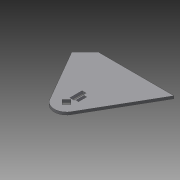
# Autodesk Inventor part: Frame_Lower_Plate_Top
Saved by Autodesk Inventor 2014 (Build 180170000, 170)
## iProperties
Created: 2014-08-25
Part Number: Frame_Lower_Plate_Top
Material: Generic
Document SubType Name: Modeling
Designer: ThatOtherGuy
Density: 1 g/cm^3
Appearance: Default
Author: ThatOtherGuy
Autodesk Inventor part; units mm, degrees
ref_plane "YZ Plane" through (0, 0, 0) normal (1, 0, 0) x (0, 1, 0)
ref_plane "XZ Plane" through (0, 0, 0) normal (0, 1, 0) x (-1, 0, 0)
ref_plane "XY Plane" through (0, 0, 0) normal (0, 0, 1) x (1, 0, 0)
sketch "Sketch1" plane through (0, 0, 0) normal (0, 0, 1) x (1, 0, 0)
  line L0 (-10.6066, 0) -> (0, 10.6066)
  line L1 (0, 10.6066) -> (10.6066, 0)
  line L2 (10.6066, 0) -> (0, -10.6066)
  line L3 (0, -10.6066) -> (-10.6066, 0)
  arc A0 (-25.9808, -15) -> (25.9808, -15) centre (0, 0) ccw
  line L4 (118.3568, 145) -> (-118.3568, 145)
  line L5 (7.5, 35.6066) -> (13.85, 35.6066)
  line L6 (13.85, 35.6066) -> (13.85, 15.6066)
  line L7 (13.85, 15.6066) -> (7.5, 15.6066)
  line L8 (7.5, 15.6066) -> (7.5, 35.6066)
  line L9 (-5, 43.1066) -> (5, 43.1066)
  line L10 (5, 43.1066) -> (5, 13.1066)
  line L11 (5, 13.1066) -> (-5, 13.1066)
  line L12 (-5, 13.1066) -> (-5, 43.1066)
  line L13 (118.3568, 145) -> (25.9808, -15)
  line L14 (-25.9808, -15) -> (-118.3568, 145)
  point P0 (0, 13.1066)
  dimension "d0" = 15
  dimension "d4" = 30
  dimension "d6" = 6.35
  dimension "d7" = 20
  dimension "d8" = 5
  dimension "d16" = 10
  dimension "d17" = 2.5
  dimension "d18" = 2.5
  dimension "d19" = 30
  dimension "d23" = 60
  dimension "d24" = 175
  constraints: 30 end point, 4 equal length, 4 parallel, 3 horizontal, 3 perpendicular, 3 vertical alignment, 2 coincident, 2 point on circle, 2 tangent, 1 centre point, 1 horizontal alignment, 1 midpoint
  measures "d0" distance of L0.start L0.end
  measures "d4" radius of A0
  measures "d6" distance of L5.start L5.end
  measures "d7" distance of L5.end L6.end
  measures "d8" distance from line of L7 L0.end
  measures "d16" distance of L10.end L11.end
  measures "d17" distance between parallel lines of L8 L10
  measures "d18" distance from line of L0.end L11
  measures "d19" distance of L11.end L9.start
  measures "d23" angle of L14 L13
extrude "Extrusion1" add sketch "Sketch1" along normal blind 6.35
body "Solid1"
